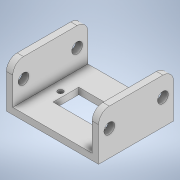
# Autodesk Inventor part: 8
Saved by Autodesk Inventor 2021 (Build 250183000, 183)
## iProperties
Created: 2021-03-30
Part Number: 8
Material: Genérico
Document SubType Name: Modeling
Designer: diego
Density: 1 g/cm^3
Appearance: Valor por defecto
Author: diego
Autodesk Inventor part; units mm, degrees
ref_plane "YZ Plane" through (0, 0, 0) normal (1, 0, 0) x (0, 1, 0)
ref_plane "XZ Plane" through (0, 0, 0) normal (0, 1, 0) x (-1, 0, 0)
ref_plane "XY Plane" through (0, 0, 0) normal (0, 0, 1) x (1, 0, 0)
sketch "Boceto1" plane through (0, 0, 0) normal (0, 0, 1) x (1, 0, 0)
  line L0 (0, 0) -> (43, 0)
  line L1 (43, 0) -> (43, 21)
  line L2 (43, 21) -> (40, 21)
  line L3 (40, 21) -> (40, 3)
  line L4 (40, 3) -> (3, 3)
  line L5 (3, 3) -> (3, 21)
  line L6 (3, 21) -> (0, 21)
  line L7 (0, 21) -> (0, 0)
  constraints: 16 end point, 4 perpendicular, 2 horizontal, 2 vertical
extrude "Extrusión1" add sketch "Boceto1" against normal blind 35
fillet "Empalme1" radius 5 4 edges at (1.5, 21, 0) (1.5, 21, -35) (41.5, 21, 0) (41.5, 21, -35)
sketch "Boceto2" plane through (43, 0, 0) normal (1, 0, 0) x (0, 0, -1)
  arc A0 (5, 21) -> (0, 16) centre (5, 16) ccw projected
  circle A1 centre (5, 12) radius 2.5
  circle A2 centre (30, 12) radius 2.5
  point P0 (0, 0)
  constraints: 2 centre point
hole "Agujero1" at (43, 12, -5) at (43, 12, -30) direction (-1, 0, 0) diameter 5 end through all
sketch "Boceto3" plane through (3, 3, 0) normal (0, 1, 0) x (1, 0, 0)
  line L0 (7.25, 23.5) -> (29.75, 23.5)
  line L1 (29.75, 23.5) -> (29.75, 11.5)
  line L2 (29.75, 11.5) -> (7.25, 11.5)
  line L3 (7.25, 11.5) -> (7.25, 23.5)
  point P0 (-3, 0)
  point P1 (0, 35)
  constraints: 8 end point, 2 perpendicular, 1 horizontal
extrude "Extrusión2" cut sketch "Boceto3" against normal blind 35
sketch "Boceto4" plane through (3, 3, 0) normal (0, 1, 0) x (1, 0, 0)
  circle A0 centre (32.25, 17.5) radius 1.25
  circle A1 centre (4.75, 17.5) radius 1.25
  point P0 (-3, 0)
  constraints: 2 centre point
hole "Agujero2" at (7.75, 3, -17.5) at (35.25, 3, -17.5) direction (0, -1, 0) diameter 2.5 end through all
